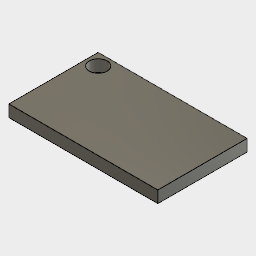
L8-PE-01 (Autodesk Fusion 360 design; units mm, degrees)
Autodesk Fusion 360 part; units mm, degrees
sketch "Sketch1" plane through (0, 0, 0) normal (0, 1, 0) x (1, 0, 0)
  line L0 (-62.5, 37.5) -> (62.5, 37.5)
  line L1 (62.5, 37.5) -> (62.5, -37.5)
  line L2 (62.5, -37.5) -> (-62.5, -37.5)
  line L3 (-62.5, -37.5) -> (-62.5, 37.5)
  line L4 (-62.5, 37.5) -> (62.5, -37.5) construction
  line L5 (62.5, 37.5) -> (-62.5, -37.5) construction
  dimension "d1" = 125
  dimension "d2" = 75
  measures "d1" distance of L1.end L2.end
  measures "d2" distance of L0.end L1.end
extrude "Extrude1" add sketch "Sketch1" along normal blind 10
sketch "Sketch2" plane through (0, 10, 0) normal (0, 1, 0) x (-1, 0, 0)
  line L0 (62.5, 37.5) -> (-62.5, 37.5)
  line L1 (-62.5, 37.5) -> (-62.5, -37.5)
  line L2 (-62.5, -37.5) -> (62.5, -37.5)
  line L3 (62.5, -37.5) -> (62.5, 37.5)
  circle A0 centre (52.5, -27.5) radius 7.5
  dimension "d5" = 15
  dimension "d6" = 10
  dimension "d7" = 10
  measures "d5" diameter of A0
  measures "d6" distance of L2 A0.centre
  measures "d7" distance of L3 A0.centre
extrude "Extrude2" cut sketch "Sketch2" against normal through all contours A0
